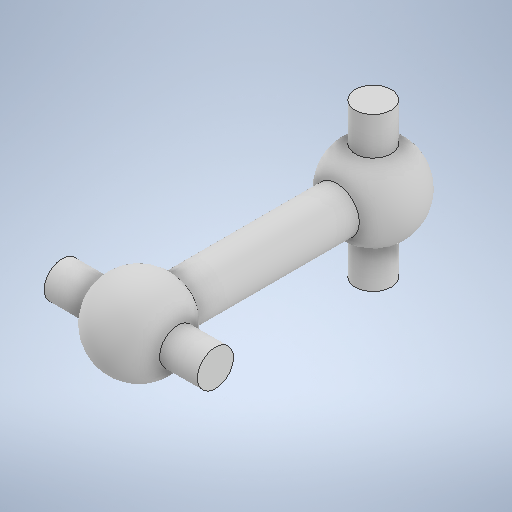
# Autodesk Inventor part: wal
Saved by Autodesk Inventor 2025.2 (Build 292293000, 293)
## iProperties
Created: 2025-05-31
Part Number: wal
Material: Ogólny
Document SubType Name: Modeling
Designer: janla
Density: 1 g/cm^3
Appearance: Domyślna
Author: janla
Autodesk Inventor part; units mm, degrees
ref_plane "YZ Plane" through (0, 0, 0) normal (1, 0, 0) x (0, 1, 0)
ref_plane "XZ Plane" through (0, 0, 0) normal (0, 1, 0) x (-1, 0, 0)
ref_plane "XY Plane" through (0, 0, 0) normal (0, 0, 1) x (1, 0, 0)
sketch "Szkic1" plane through (0, 0, 0) normal (0, 1, 0) x (-1, 0, 0)
  arc A0 (-4.75, 0) -> (4.75, 0) centre (0, 0) ccw
  line L0 (4.75, 0) -> (-4.75, 0)
  dimension "d0" = 9.5
  constraints: 2 end point, 2 point on circle, 1 centre point, 1 coincident, 1 horizontal
  measures "d0" diameter of A0
revolve "Obrót1" add sketch "Szkic1" angle 360 about axis through (-4.75, 0, 0) along (1, 0, 0)
sketch "Szkic2" plane through (0, 0, 0) normal (0, 1, 0) x (-1, 0, 0)
  line L0 (0, 0) -> (0, -26)
  arc A0 (-4.75, -26) -> (4.75, -26) centre (0, -26) ccw
  line L1 (-4.75, -26) -> (4.75, -26)
  dimension "d2" = 26
  dimension "d3" = 9.5
  constraints: 4 end point, 2 point on circle, 1 centre point, 1 coincident, 1 horizontal, 1 vertical
  measures "d2" distance of L0.start L0.end
  measures "d3" diameter of A0
revolve "Obrót2" add sketch "Szkic2" angle 360 about axis through (4.75, 0, -26) along (-1, 0, 0)
sketch "Szkic3" plane through (0, 0, 0) normal (0, 0, 1) x (1, 0, 0)
  circle A0 centre (0, 0) radius 2.5
  dimension "d5" = 5
  constraints: 1 centre point, 1 coincident
  measures "d5" diameter of A0
extrude "Wyciągnięcie proste1" add sketch "Szkic3" against normal blind 26
sketch "Szkic4" plane through (0, 0, 0) normal (1, 0, 0) x (0, 1, 0)
  circle A0 centre (0, 0) radius 2
  circle A1 centre (0, 0) radius 2
  dimension "d8" = 4
  dimension "d11" = 4
  constraints: 2 centre point, 2 coincident
  measures "d8" diameter of A0
  measures "d11" diameter of A1
extrude "Wyciągnięcie proste2" add sketch "Szkic4" along normal mid plane 17
sketch "Szkic5" plane through (0, 0, 0) normal (0, 1, 0) x (-1, 0, 0)
  line L0 (0, 0) -> (0, -26)
  circle A0 centre (0, -26) radius 2
  dimension "d12" = 26
  dimension "d13" = 4
  constraints: 2 end point, 1 centre point, 1 coincident, 1 vertical
  measures "d12" distance of L0.start L0.end
  measures "d13" diameter of A0
extrude "Wyciągnięcie proste3" add sketch "Szkic5" along normal mid plane 17
